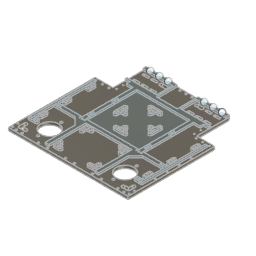
Chassis-200x200x8mm (Autodesk Fusion 360 design; units mm, degrees)
part number: 2026-04-02-11-57-34-569
Autodesk Fusion 360 part; units mm, degrees
(part 1 of 2)
sketch "Sketch1" plane through (0, 0, 0) normal (0, 0, 1) x (1, 0, 0)
  line L0 (67.5, 102.5) -> (-72.5, 102.5)
  line L1 (-102.5, 47.5) -> (-102.5, -97.5)
  line L2 (-102.5, -97.5) -> (97.5, -97.5)
  line L3 (97.5, -97.5) -> (97.5, 47.5)
  line L4 (-72.5, 102.5) -> (-72.5, 52.5)
  line L5 (67.5, 102.5) -> (67.5, 52.5)
  line L6 (-65.9, 77.6) -> (-58.1, 77.6)
  line L7 (-65.9, 74.4) -> (-58.1, 74.4)
  line L8 (-51.9, 77.6) -> (-44.1, 77.6)
  line L9 (-51.9, 74.4) -> (-44.1, 74.4)
  arc A0 (-65.9, 77.6) -> (-65.9, 74.4) centre (-65.9, 76) ccw
  arc A1 (-58.1, 74.4) -> (-58.1, 77.6) centre (-58.1, 76) ccw
  arc A2 (-51.9, 77.6) -> (-51.9, 74.4) centre (-51.9, 76) ccw
  arc A3 (-44.1, 74.4) -> (-44.1, 77.6) centre (-44.1, 76) ccw
  arc A4 (-44.1, 90.4) -> (-44.1, 93.6) centre (-44.1, 92) ccw
  line L10 (-51.9, 90.4) -> (-44.1, 90.4)
  line L11 (-51.9, 93.6) -> (-44.1, 93.6)
  arc A5 (-51.9, 93.6) -> (-51.9, 90.4) centre (-51.9, 92) ccw
  line L12 (-65.9, 93.6) -> (-58.1, 93.6)
  arc A6 (-58.1, 90.4) -> (-58.1, 93.6) centre (-58.1, 92) ccw
  line L13 (-65.9, 90.4) -> (-58.1, 90.4)
  arc A7 (-65.9, 93.6) -> (-65.9, 90.4) centre (-65.9, 92) ccw
  line L14 (39.1, 74.4) -> (46.9, 74.4)
  arc A8 (39.1, 77.6) -> (39.1, 74.4) centre (39.1, 76) ccw
  line L15 (39.1, 77.6) -> (46.9, 77.6)
  arc A9 (46.9, 74.4) -> (46.9, 77.6) centre (46.9, 76) ccw
  arc A10 (53.1, 77.6) -> (53.1, 74.4) centre (53.1, 76) ccw
  line L16 (53.1, 74.4) -> (60.9, 74.4)
  line L17 (53.1, 77.6) -> (60.9, 77.6)
  arc A11 (60.9, 74.4) -> (60.9, 77.6) centre (60.9, 76) ccw
  arc A12 (39.1, 93.6) -> (39.1, 90.4) centre (39.1, 92) ccw
  line L18 (39.1, 90.4) -> (46.9, 90.4)
  line L19 (39.1, 93.6) -> (46.9, 93.6)
  arc A13 (46.9, 90.4) -> (46.9, 93.6) centre (46.9, 92) ccw
  line L20 (53.1, 90.4) -> (60.9, 90.4)
  arc A14 (53.1, 93.6) -> (53.1, 90.4) centre (53.1, 92) ccw
  line L21 (53.1, 93.6) -> (60.9, 93.6)
  arc A15 (60.9, 90.4) -> (60.9, 93.6) centre (60.9, 92) ccw
  arc A16 (-37.9, 77.6) -> (-37.9, 74.4) centre (-37.9, 76) ccw
  line L22 (-37.9, 77.6) -> (-30.1, 77.6)
  arc A17 (-30.1, 74.4) -> (-30.1, 77.6) centre (-30.1, 76) ccw
  line L23 (-37.9, 74.4) -> (-30.1, 74.4)
  line L24 (25.1, 77.6) -> (32.9, 77.6)
  arc A18 (32.9, 74.4) -> (32.9, 77.6) centre (32.9, 76) ccw
  line L25 (25.1, 74.4) -> (32.9, 74.4)
  arc A19 (25.1, 77.6) -> (25.1, 74.4) centre (25.1, 76) ccw
  line L26 (-36.9, 94.551) -> (-28.0006, 94.551)
  line L27 (-36.9006, 89.451) -> (-28.0006, 89.451)
  arc A20 (-36.9, 94.551) -> (-36.9006, 89.451) centre (-36.9006, 92.001) ccw
  arc A21 (-28.0006, 89.451) -> (-28.0006, 94.551) centre (-28.0006, 92.001) ccw
  line L28 (23, 94.551) -> (31.8994, 94.551)
  arc A22 (23, 94.551) -> (22.9994, 89.451) centre (22.9994, 92.001) ccw
  line L29 (22.9994, 89.451) -> (31.8994, 89.451)
  arc A23 (31.8994, 89.451) -> (31.8994, 94.551) centre (31.8994, 92.001) ccw
  line L30 (-72.5, 52.5) -> (-72.5, 47.5)
  line L31 (-72.5, 47.5) -> (-102.5, 47.5)
  line L32 (67.5, 52.5) -> (67.5, 47.5)
  line L33 (67.5, 47.5) -> (97.5, 47.5)
  line L34 (97.5, -97.5) -> (-102.5, -97.5)
  line L35 (-102.5, -97.5) -> (-102.5, -92.5)
  line L36 (97.5, -92.5) -> (97.5, -97.5)
  line L37 (75.5, -90.5) -> (45.5, -90.5)
  line L38 (45.5, -90.5) -> (45.5, -40.5)
  line L39 (45.5, -40.5) -> (75.5, -40.5)
  line L40 (75.5, -40.5) -> (75.5, -90.5)
  line L41 (-80.5, -90.5) -> (-50.5, -90.5)
  line L42 (-50.5, -90.5) -> (-50.5, -40.5)
  line L43 (-50.5, -40.5) -> (-80.5, -40.5)
  line L44 (-80.5, -40.5) -> (-80.5, -90.5)
  line L45 (79, -84.449) -> (85.3494, -84.449)
  line L46 (78.9994, -89.549) -> (87.8994, -89.549)
  arc A24 (87.8994, -89.549) -> (90.4494, -86.9852) centre (87.8994, -86.999) ccw
  arc A25 (79, -84.449) -> (78.9994, -89.549) centre (78.9994, -86.999) ccw
  line L47 (-93.0006, -89.549) -> (-84.1006, -89.549)
  line L48 (-90.4506, -84.449) -> (-84.1006, -84.449)
  arc A26 (-84.1006, -89.549) -> (-84.1006, -84.449) centre (-84.1006, -86.999) ccw
  arc A27 (-95.5506, -86.985) -> (-93.0006, -89.549) centre (-93.0006, -86.999) ccw
  line L49 (90.4494, -86.9991) -> (90.4494, -78.099)
  arc A28 (87.8854, -89.549) -> (90.4494, -86.9991) centre (87.8994, -86.9991) ccw
  line L50 (85.3494, -84.449) -> (85.3494, -78.099)
  arc A29 (90.4494, -78.099) -> (85.3494, -78.099) centre (87.8994, -78.099) ccw
  line L51 (-95.5506, -78.099) -> (-95.5506, -86.9991)
  arc A30 (-90.4506, -78.0996) -> (-95.5506, -78.099) centre (-93.0006, -78.099) ccw
  line L52 (-90.4506, -78.0996) -> (-90.4506, -84.449)
  arc A31 (-95.5506, -86.9991) -> (-92.9866, -89.549) centre (-93.0006, -86.9991) ccw
  circle A32 centre (-65.5, -65.5) radius 15
  circle A33 centre (-65.5, -85) radius 2
  circle A34 centre (-65.5, -46) radius 2
  circle A35 centre (60.5, -85) radius 2
  circle A36 centre (60.5, -65.5) radius 15
  circle A37 centre (60.5, -46) radius 2
  line L53 (75.5, -80.5) -> (45.5, -80.5)
  line L54 (75.5, -50.5) -> (45.5, -50.5)
  line L55 (-50.5, -80.5) -> (-80.5, -80.5)
  line L56 (-50.5, -50.5) -> (-80.5, -50.5)
  line L57 (-70.5, 67.5) -> (-72.5, 67.5)
  line L58 (-70.5, 67.5) -> (-64.5, 67.5)
  line L59 (-64.5, 67.5) -> (-62.5, 67.5)
  circle A38 centre (-67.5, 59.5) radius 1.15
  circle A39 centre (-67.5, 48.623) radius 1.15
  circle A40 centre (-67.5, 48.623) radius 1.15
  circle A41 centre (-67.5, 59.5) radius 1.15
  line L60 (-64.5, 67.5) -> (-62.5, 67.5)
  line L61 (-70.5, 67.5) -> (-64.5, 67.5)
  line L62 (-70.5, 67.5) -> (-72.5, 67.5)
  circle A42 centre (62.5, 48.623) radius 1.15
  circle A43 centre (62.5, 59.5) radius 1.15
  line L63 (65.5, 67.5) -> (67.5, 67.5)
  line L64 (59.5, 67.5) -> (65.5, 67.5)
  line L65 (59.5, 67.5) -> (57.5, 67.5)
  circle A44 centre (-86.5, 43.5) radius 1.35
  circle A45 centre (-97.5, 43.5) radius 1.35
  circle A46 centre (-75.5, 43.5) radius 1.35
  circle A47 centre (92.5, 43.5) radius 1.35
  circle A48 centre (70.5, 43.5) radius 1.35
  circle A49 centre (81.5, 43.5) radius 1.35
  line L66 (-2.5, -97.5) -> (-2.5, 102.5)
  circle A50 centre (2.5, 94.5) radius 1.6
  dimension "d64" = 200
  dimension "d104" = 6
  dimension "d107" = 2
  dimension "d110" = 6
  dimension "d111" = 2
  dimension "d121" = 2.7
  dimension "d122" = 2.7
  dimension "d165" = 50
  dimension "d166" = 10
  dimension "d167" = 30
  dimension "d181" = 2.3
  dimension "d237" = 8.9001
  dimension "d238" = 5.1
  constraint horizontal L0
  constraint perpendicular L0 L1
  constraint parallel L0 L2
  constraint parallel L1 L3
  constraint vertical L4
  constraint vertical L5
  constraint tangent L6 A1
  constraint tangent L7 A1
  constraint tangent L8 A3
  constraint tangent L9 A3
  constraint tangent L12 A6
  constraint tangent A6 L13
  constraint tangent A4 L11
  constraint tangent A4 L10
  constraint tangent L15 A9
  constraint tangent L14 A9
  constraint tangent L17 A11
  constraint tangent L16 A11
  constraint tangent L19 A13
  constraint tangent L18 A13
  constraint tangent L21 A15
  constraint tangent L20 A15
  constraint tangent L22 A17
  constraint tangent A17 L23
  constraint tangent L24 A18
  constraint tangent A18 L25
  constraint tangent L26 A21
  constraint horizontal L26
  constraint tangent L27 A21
  constraint tangent L28 A23
  constraint horizontal L28
  constraint tangent L29 A23
  constraint perpendicular L1 L31
  constraint perpendicular L3 L33
  constraint horizontal L34
  constraint vertical L35
  constraint vertical L36
  constraint horizontal L37
  constraint vertical L38
  constraint horizontal L39
  constraint vertical L40
  constraint horizontal L41
  constraint vertical L42
  constraint horizontal L43
  constraint vertical L44
  constraint tangent L45 A24
  constraint tangent L46 A24
  constraint tangent L48 A26
  constraint tangent L47 A26
  constraint tangent L50 A29
  constraint tangent L49 A29
  constraint tangent L52 A31
  constraint tangent L51 A31
  constraint coincident L47 A31.end
  constraint coincident L51 A27.start
  constraint coincident L46 A28.start
  constraint coincident L49 A24.end
  constraint coincident L40 L53.start
  constraint perpendicular L38 L53
  constraint coincident L40 L54.start
  constraint coincident L38 L54.end
  constraint perpendicular L38 L54
  constraint coincident L4 L57.end
  constraint perpendicular L4 L57
  constraint parallel L58 L59
  constraint parallel L60 L61
  constraint midpoint L34 L66.start
  constraint midpoint L0 L66.end
  constraint perpendicular L0 L66
  measures "d64" distance of L2.end L1.end
  measures "d104" distance of L57.start L58.end
  measures "d107" distance of L58.end L59.end
  measures "d110" distance of L57.start L58.end
  measures "d111" distance of L59.end L58.end
  measures "d121" diameter of A46
  measures "d122" diameter of A47
  measures "d165" distance of L41 L43
  measures "d166" distance of L43 L56
  measures "d167" distance of L42 L44
  measures "d181" diameter of A39
  measures "d237" distance of A22.centre A23.centre
  measures "d238" distance of L28 L29
extrude "Extrude1" add sketch "Sketch1" along normal blind 5 contours L0 L2 L3 L5 L32 L33 L34 L36 L66 | L0 L1 L2 L4 L30 L31 L34 L35 L66 | L37 L38 L40 L53 | L40 A36 L53 | L38 A36 L53 | L40 A36 L54 | L38 A36 L54 | L38 L39 L40 L54 | L41 L42 L44 L55 | L44 A32 L55 | L42 A32 L55 | L44 A32 L56 | L42 A32 L56 | L42 L43 L44 L56 | A50 makes body 1
fillet "Fillet1" radius 3 1 edges at (-2.5, 102.5, 0) on bodies 1
sketch "Sketch2" plane through (0, 0, 5) normal (0, 0, 1) x (-1, 0, 0)
  line L0 (-67.5, -102.5) -> (72.5, -102.5)
  line L1 (72.5, -102.5) -> (72.5, -47.5)
  line L2 (102.5, -47.5) -> (102.5, 97.5)
  line L3 (102.5, 97.5) -> (-97.5, 97.5)
  line L4 (-97.5, 97.5) -> (-97.5, -47.5)
  line L5 (-67.5, -47.5) -> (-67.5, -102.5)
  line L6 (72.5, -102.5) -> (22.5, -102.5)
  line L7 (22.5, -102.5) -> (22.5, -97.5)
  line L8 (22.5, -97.5) -> (72.5, -97.5)
  line L9 (72.5, -97.5) -> (72.5, -102.5)
  line L10 (27.5, -67.5) -> (72.5, -67.5)
  line L11 (72.5, -67.5) -> (72.5, -70.5)
  line L12 (-22.5, -67.5) -> (-67.5, -67.5)
  line L13 (-67.5, -67.5) -> (-67.5, -70.5)
  arc A0 (65.9, -77.6) -> (65.9, -74.4) centre (65.9, -76) ccw
  line L14 (65.9, -77.6) -> (58.1, -77.6)
  arc A1 (58.1, -74.4) -> (58.1, -77.6) centre (58.1, -76) ccw
  line L15 (58.1, -74.4) -> (65.9, -74.4)
  arc A2 (-53.1, -93.6) -> (-53.1, -90.4) centre (-53.1, -92) ccw
  line L16 (-53.1, -93.6) -> (-60.9, -93.6)
  arc A3 (-60.9, -90.4) -> (-60.9, -93.6) centre (-60.9, -92) ccw
  line L17 (-60.9, -90.4) -> (-53.1, -90.4)
  arc A4 (65.9, -93.6) -> (65.9, -90.4) centre (65.9, -92) ccw
  line L18 (65.9, -93.6) -> (58.1, -93.6)
  arc A5 (58.1, -90.4) -> (58.1, -93.6) centre (58.1, -92) ccw
  line L19 (58.1, -90.4) -> (65.9, -90.4)
  arc A6 (-39.1, -77.6) -> (-39.1, -74.4) centre (-39.1, -76) ccw
  line L20 (-39.1, -77.6) -> (-46.9, -77.6)
  arc A7 (-46.9, -74.4) -> (-46.9, -77.6) centre (-46.9, -76) ccw
  line L21 (-46.9, -74.4) -> (-39.1, -74.4)
  arc A8 (-53.1, -77.6) -> (-53.1, -74.4) centre (-53.1, -76) ccw
  line L22 (-53.1, -77.6) -> (-60.9, -77.6)
  arc A9 (-60.9, -74.4) -> (-60.9, -77.6) centre (-60.9, -76) ccw
  line L23 (-60.9, -74.4) -> (-53.1, -74.4)
  arc A10 (51.9, -93.6) -> (51.9, -90.4) centre (51.9, -92) ccw
  line L24 (51.9, -93.6) -> (44.1, -93.6)
  arc A11 (44.1, -90.4) -> (44.1, -93.6) centre (44.1, -92) ccw
  line L25 (44.1, -90.4) -> (51.9, -90.4)
  arc A12 (51.9, -77.6) -> (51.9, -74.4) centre (51.9, -76) ccw
  line L26 (51.9, -77.6) -> (44.1, -77.6)
  arc A13 (44.1, -74.4) -> (44.1, -77.6) centre (44.1, -76) ccw
  line L27 (44.1, -74.4) -> (51.9, -74.4)
  arc A14 (-39.1, -93.6) -> (-39.1, -90.4) centre (-39.1, -92) ccw
  line L28 (-39.1, -93.6) -> (-46.9, -93.6)
  arc A15 (-46.9, -90.4) -> (-46.9, -93.6) centre (-46.9, -92) ccw
  line L29 (-46.9, -90.4) -> (-39.1, -90.4)
  arc A16 (-25.1, -77.6) -> (-25.1, -74.4) centre (-25.1, -76) ccw
  line L30 (-25.1, -77.6) -> (-32.9, -77.6)
  arc A17 (-32.9, -74.4) -> (-32.9, -77.6) centre (-32.9, -76) ccw
  line L31 (-32.9, -74.4) -> (-25.1, -74.4)
  arc A18 (37.9, -77.6) -> (37.9, -74.4) centre (37.9, -76) ccw
  line L32 (37.9, -77.6) -> (30.1, -77.6)
  arc A19 (30.1, -74.4) -> (30.1, -77.6) centre (30.1, -76) ccw
  line L33 (30.1, -74.4) -> (37.9, -74.4)
  line L34 (-67.5, -102.5) -> (-17.5, -102.5)
  line L35 (-17.5, -102.5) -> (-17.5, -97.5)
  line L36 (-17.5, -97.5) -> (-67.5, -97.5)
  line L37 (-67.5, -97.5) -> (-67.5, -102.5)
  line L38 (72.5, -47.5) -> (102.5, -47.5)
  line L39 (-97.5, -47.5) -> (-67.5, -47.5)
  arc A20 (-23, -94.551) -> (-22.9994, -89.451) centre (-22.9994, -92.001) ccw
  line L40 (-23, -94.551) -> (-31.8994, -94.551)
  arc A21 (-31.8994, -89.451) -> (-31.8994, -94.551) centre (-31.8994, -92.001) ccw
  line L41 (-31.8994, -89.451) -> (-22.9994, -89.451)
  arc A22 (36.9, -94.551) -> (36.9006, -89.451) centre (36.9006, -92.001) ccw
  line L42 (36.9, -94.551) -> (28.0006, -94.551)
  arc A23 (28.0006, -89.451) -> (28.0006, -94.551) centre (28.0006, -92.001) ccw
  line L43 (28.0006, -89.451) -> (36.9006, -89.451)
  circle A24 centre (65.5, 85) radius 2
  circle A25 centre (-60.5, 46) radius 2
  circle A26 centre (-60.5, 65.5) radius 15
  arc A27 (-79, 84.449) -> (-78.9994, 89.549) centre (-78.9994, 86.999) ccw
  line L44 (-79, 84.449) -> (-85.3494, 84.449)
  line L45 (-85.3494, 84.449) -> (-85.3494, 78.099)
  arc A28 (-90.4494, 78.099) -> (-85.3494, 78.099) centre (-87.8994, 78.099) ccw
  line L46 (-90.4494, 78.099) -> (-90.4494, 86.9852)
  arc A29 (-89.7213, 88.7832) -> (-90.4494, 86.9852) centre (-87.8994, 86.999) ccw
  arc A30 (-87.8854, 89.549) -> (-89.7213, 88.7832) centre (-87.8994, 86.9991) ccw
  line L47 (-87.8854, 89.549) -> (-78.9994, 89.549)
  circle A31 centre (-60.5, 85) radius 2
  circle A32 centre (65.5, 46) radius 2
  circle A33 centre (65.5, 65.5) radius 15
  arc A34 (90.4506, 78.0996) -> (95.5506, 78.099) centre (93.0006, 78.099) ccw
  line L48 (90.4506, 78.0996) -> (90.4506, 84.449)
  line L49 (90.4506, 84.449) -> (84.1006, 84.449)
  arc A35 (84.1006, 89.549) -> (84.1006, 84.449) centre (84.1006, 86.999) ccw
  line L50 (84.1006, 89.549) -> (92.9866, 89.549)
  arc A36 (94.8063, 88.7996) -> (92.9866, 89.549) centre (93.0006, 86.9991) ccw
  arc A37 (95.5506, 86.985) -> (94.8063, 88.7996) centre (93.0006, 86.999) ccw
  line L51 (95.5506, 86.985) -> (95.5506, 78.099)
  circle A38 centre (90, -32) radius 1.15
  circle A39 centre (90, 8) radius 1.15
  circle A40 centre (67.5, -59.5) radius 1.15
  circle A41 centre (67.5, -48.623) radius 1.15
  circle A42 centre (-62.5, -48.623) radius 1.15
  circle A43 centre (-62.5, -59.5) radius 1.15
  circle A44 centre (75.5, -43.5) radius 1.35
  circle A45 centre (97.5, -43.5) radius 1.35
  circle A46 centre (86.5, -43.5) radius 1.35
  circle A47 centre (-81.5, -43.5) radius 1.35
  circle A48 centre (-92.5, -43.5) radius 1.35
  circle A49 centre (-70.5, -43.5) radius 1.35
  line L52 (72.5, -67.5) -> (64.5, -67.5)
  line L53 (64.5, -67.5) -> (64.5, -40.6151)
  line L54 (64.5, -40.6151) -> (102.5, -40.6151)
  line L55 (-67.5, -67.5) -> (-59.5, -67.5)
  line L56 (-59.5, -67.5) -> (-59.5, -40.6151)
  line L57 (-59.5, -40.6151) -> (-97.5, -40.6151)
  circle A50 centre (90, -32) radius 1.15
  circle A51 centre (90, -24) radius 1.15
  circle A52 centre (90, 16) radius 1.15
  arc A53 (87.0072, -31.7917) -> (93, -32) centre (90, -32) ccw
  arc A54 (87.0072, -31.7917) -> (93, -32) centre (90, -32) ccw
  arc A55 (93, -24) -> (87, -24.0028) centre (90, -24) ccw
  line L58 (93, -32) -> (93, -24)
  line L59 (87.0072, -31.7917) -> (87, -24.0028)
  circle A56 centre (89.9963, -28) radius 1.4
  line L60 (87.0106, 8.0515) -> (87, 15.996)
  line L61 (93, 8) -> (93, 16)
  circle A57 centre (90, 12) radius 1.4
  arc A58 (87.0104, 8.2491) -> (93, 8) centre (90, 8) ccw
  arc A59 (87.0104, 8.2491) -> (93, 8) centre (90, 8) ccw
  arc A60 (93, 16) -> (87, 15.996) centre (90, 16) ccw
  line L62 (87.0072, -31.7917) -> (87, -24.0028)
  arc A61 (87.0072, -31.7917) -> (93, -32) centre (90, -32) ccw
  line L63 (93, -32) -> (93, -24)
  arc A62 (93, -24) -> (87, -24.0028) centre (90, -24) ccw
  circle A63 centre (90, -24) radius 1.15
  circle A64 centre (89.9963, -28) radius 1.4
  circle A65 centre (90, -32) radius 1.15
  arc A66 (87.0104, 8.2491) -> (93, 8) centre (90, 8) ccw
  line L64 (93, 8) -> (93, 16)
  circle A67 centre (90, 16) radius 1.15
  circle A68 centre (90, 12) radius 1.4
  circle A69 centre (90, 8) radius 1.15
  arc A70 (93, 16) -> (87, 15.996) centre (90, 16) ccw
  line L65 (87.0106, 8.0515) -> (87, 15.996)
  line L66 (47.0072, -31.7917) -> (47, -24.0028)
  arc A71 (47.0072, -31.7917) -> (53, -32) centre (50, -32) ccw
  line L67 (53, -32) -> (53, -24)
  arc A72 (53, -24) -> (47, -24.0028) centre (50, -24) ccw
  circle A73 centre (50, -24) radius 1.15
  circle A74 centre (49.9963, -28) radius 1.4
  circle A75 centre (50, -32) radius 1.15
  line L68 (47.0106, 8.0515) -> (47, 15.996)
  arc A76 (47.0104, 8.2491) -> (53, 8) centre (50, 8) ccw
  line L69 (53, 8) -> (53, 16)
  arc A77 (53, 16) -> (47, 15.996) centre (50, 16) ccw
  circle A78 centre (50, 8) radius 1.15
  circle A79 centre (50, 12) radius 1.4
  circle A80 centre (50, 16) radius 1.15
  line L70 (-87.9928, -31.7917) -> (-88, -24.0028)
  arc A81 (-87.9928, -31.7917) -> (-82, -32) centre (-85, -32) ccw
  line L71 (-82, -32) -> (-82, -24)
  arc A82 (-82, -24) -> (-88, -24.0028) centre (-85, -24) ccw
  circle A83 centre (-85, -24) radius 1.15
  circle A84 centre (-85.0037, -28) radius 1.4
  circle A85 centre (-85, -32) radius 1.15
  line L72 (-87.9894, 8.0515) -> (-88, 15.996)
  arc A86 (-87.9896, 8.2491) -> (-82, 8) centre (-85, 8) ccw
  line L73 (-82, 8) -> (-82, 16)
  arc A87 (-82, 16) -> (-88, 15.996) centre (-85, 16) ccw
  circle A88 centre (-85, 8) radius 1.15
  circle A89 centre (-85, 12) radius 1.4
  circle A90 centre (-85, 16) radius 1.15
  arc A91 (-47.9928, -31.7917) -> (-42, -32) centre (-45, -32) ccw
  circle A92 centre (-45, -32) radius 1.15
  line L74 (-42, -32) -> (-42, -24)
  line L75 (-47.9928, -31.7917) -> (-48, -24.0028)
  circle A93 centre (-45.0037, -28) radius 1.4
  circle A94 centre (-45, -24) radius 1.15
  arc A95 (-42, -24) -> (-48, -24.0028) centre (-45, -24) ccw
  arc A96 (-47.9896, 8.2491) -> (-42, 8) centre (-45, 8) ccw
  line L76 (-47.9894, 8.0515) -> (-48, 15.996)
  arc A97 (-42, 16) -> (-48, 15.996) centre (-45, 16) ccw
  line L77 (-42, 8) -> (-42, 16)
  circle A98 centre (-45, 12) radius 1.4
  circle A99 centre (-45, 16) radius 1.15
  circle A100 centre (-45, 8) radius 1.15
  line L78 (-35, -59) -> (40, -59)
  line L79 (40, -59) -> (40, 21)
  line L80 (40, 21) -> (-35, 21)
  line L81 (-35, 21) -> (-35, -59)
  line L82 (64, -67.5) -> (64, -61.5)
  line L83 (64, -61.5) -> (-59, -61.5)
  line L84 (-59, -61.5) -> (-59, -67.5)
  line L85 (27.5, -67.5) -> (-22.5, -67.5)
  line L86 (102.5, -40.6151) -> (97.5, -40.6151)
  line L87 (97.5, -40.6151) -> (97.5, 91.5)
  line L88 (102.5, 97.5) -> (102.5, -40.6151)
  line L89 (-97.5, -40.6151) -> (-92.5, -40.6151)
  line L90 (-92.5, -40.6151) -> (-92.5, 91.5)
  line L91 (-97.5, 97.5) -> (-97.5, -40.6151)
  line L92 (94.5, 29.5) -> (59, 29.5)
  line L93 (47, 23.5) -> (47, -61.5)
  line L94 (47, -61.5) -> (53, -61.5)
  line L95 (53, -61.5) -> (53, 23.5)
  line L96 (-89.5, 29.5) -> (-54, 29.5)
  line L97 (-42, 23.5) -> (-42, -61.5)
  line L98 (-42, -61.5) -> (-48, -61.5)
  line L99 (-48, -61.5) -> (-48, 23.5)
  line L100 (41, 29.5) -> (-36, 29.5)
  line L101 (94.5, 23.5) -> (53, 23.5)
  line L102 (47, 23.5) -> (-42, 23.5)
  line L103 (-48, 23.5) -> (-89.5, 23.5)
  line L104 (22.5, -102.5) -> (20, -102.5)
  line L105 (20, -102.5) -> (20, -67.5)
  line L106 (20, -67.5) -> (22.5, -67.5)
  line L107 (22.5, -67.5) -> (22.5, -102.5)
  line L108 (-17.5, -102.5) -> (-15, -102.5)
  line L109 (-15, -102.5) -> (-15, -67.5)
  line L110 (-15, -67.5) -> (-17.5, -67.5)
  line L111 (-17.5, -67.5) -> (-17.5, -102.5)
  line L112 (22.5, -70.5) -> (72.5, -70.5)
  line L113 (-17.5, -70.5) -> (-67.5, -70.5)
  line L114 (97.5, 91.5) -> (-92.5, 91.5)
  line L115 (47, 41.5) -> (47, 91.5)
  line L116 (41, 29.5) -> (41, 91.5)
  line L117 (50.5, 40.5) -> (80.5, 40.5)
  line L118 (80.5, 40.5) -> (80.5, 90.5)
  line L119 (80.5, 90.5) -> (50.5, 90.5)
  line L120 (50.5, 90.5) -> (50.5, 40.5)
  line L121 (50.5, 40.5) -> (80.5, 90.5) construction
  line L122 (80.5, 40.5) -> (50.5, 90.5) construction
  line L123 (59, 29.5) -> (47, 41.5)
  line L124 (59, 29.5) -> (75.9706, 29.5) construction
  line L125 (-42, 41.5) -> (-42, 91.5)
  line L126 (-36, 91.5) -> (-36, 29.5)
  line L127 (-54, 29.5) -> (-42, 41.5)
  line L128 (87.0072, -31.7917) -> (87, -24.0028)
  arc A101 (87.0072, -31.7917) -> (93, -32) centre (90, -32) ccw
  line L129 (93, -32) -> (93, -24)
  arc A102 (93, -24) -> (87, -24.0028) centre (90, -24) ccw
  circle A103 centre (89.9963, -28) radius 1.4
  circle A104 centre (90, -32) radius 1.15
  circle A105 centre (90, -24) radius 1.15
  line L130 (87.0106, 8.0515) -> (87, 15.996)
  arc A106 (87.0104, 8.2491) -> (93, 8) centre (90, 8) ccw
  line L131 (93, 8) -> (93, 16)
  arc A107 (93, 16) -> (87, 15.996) centre (90, 16) ccw
  circle A108 centre (90, 16) radius 1.15
  circle A109 centre (90, 12) radius 1.4
  circle A110 centre (90, 8) radius 1.15
  line L132 (87.0106, 48.0515) -> (87, 55.996)
  arc A111 (87.0104, 48.2491) -> (93, 48) centre (90, 48) ccw
  line L133 (93, 48) -> (93, 56)
  circle A112 centre (90, 52) radius 1.4
  arc A113 (93, 56) -> (87, 55.996) centre (90, 56) ccw
  circle A114 centre (90, 48) radius 1.15
  circle A115 centre (90, 56) radius 1.15
  line L134 (-87.9894, 48.0515) -> (-88, 55.996)
  arc A116 (-87.9896, 48.2491) -> (-82, 48) centre (-85, 48) ccw
  line L135 (-82, 48) -> (-82, 56)
  circle A117 centre (-85, 52) radius 1.4
  arc A118 (-82, 56) -> (-88, 55.996) centre (-85, 56) ccw
  circle A119 centre (-85, 48) radius 1.15
  circle A120 centre (-85, 56) radius 1.15
  line L136 (87.0106, 8.0515) -> (87, 15.996)
  arc A121 (87.0104, 8.2491) -> (93, 8) centre (90, 8) ccw
  line L137 (93, 8) -> (93, 16)
  circle A122 centre (90, 12) radius 1.4
  arc A123 (93, 16) -> (87, 15.996) centre (90, 16) ccw
  circle A124 centre (90, 8) radius 1.15
  circle A125 centre (90, 16) radius 1.15
  line L138 (93.9776, 23.529) -> (86.0331, 23.5184)
  arc A126 (93.7799, 23.5288) -> (94.029, 29.5184) centre (94.029, 26.5184) ccw
  line L139 (94.029, 29.5184) -> (86.029, 29.5184)
  circle A127 centre (90.029, 26.5184) radius 1.4
  arc A128 (86.029, 29.5184) -> (86.0331, 23.5184) centre (86.029, 26.5184) ccw
  circle A129 centre (94.029, 26.5184) radius 1.15
  circle A130 centre (86.029, 26.5184) radius 1.15
  line L140 (87.0106, 8.0515) -> (87, 15.996)
  arc A131 (87.0104, 8.2491) -> (93, 8) centre (90, 8) ccw
  line L141 (93, 8) -> (93, 16)
  circle A132 centre (90, 12) radius 1.4
  arc A133 (93, 16) -> (87, 15.996) centre (90, 16) ccw
  circle A134 centre (90, 8) radius 1.15
  circle A135 centre (90, 16) radius 1.15
  line L142 (86, 63.5) -> (94, 63.5)
  circle A136 centre (90, 66.5) radius 1.4
  arc A137 (94, 63.5) -> (93.996, 69.5) centre (94, 66.5) ccw
  arc A138 (86.2491, 69.4896) -> (86, 63.5) centre (86, 66.5) ccw
  line L143 (86.0515, 69.4894) -> (93.996, 69.5)
  circle A139 centre (86, 66.5) radius 1.15
  circle A140 centre (94, 66.5) radius 1.15
  line L144 (46, 23.5) -> (54, 23.5)
  circle A141 centre (50, 26.5) radius 1.4
  arc A142 (54, 23.5) -> (53.996, 29.5) centre (54, 26.5) ccw
  arc A143 (46.2491, 29.4896) -> (46, 23.5) centre (46, 26.5) ccw
  line L145 (46.0515, 29.4894) -> (53.996, 29.5)
  circle A144 centre (46, 26.5) radius 1.15
  circle A145 centre (54, 26.5) radius 1.15
  line L146 (-82, 48) -> (-82, 56)
  arc A146 (-87.9896, 48.2491) -> (-82, 48) centre (-85, 48) ccw
  line L147 (-87.9894, 48.0515) -> (-88, 55.996)
  arc A147 (-82, 56) -> (-88, 55.996) centre (-85, 56) ccw
  circle A148 centre (-85, 56) radius 1.15
  circle A149 centre (-85, 52) radius 1.4
  circle A150 centre (-85, 48) radius 1.15
  line L148 (-81, 29.5) -> (-89, 29.5)
  arc A151 (-81.2491, 23.5104) -> (-81, 29.5) centre (-81, 26.5) ccw
  line L149 (-81.0515, 23.5106) -> (-88.996, 23.5)
  arc A152 (-89, 29.5) -> (-88.996, 23.5) centre (-89, 26.5) ccw
  circle A153 centre (-89, 26.5) radius 1.15
  circle A154 centre (-85, 26.5) radius 1.4
  circle A155 centre (-81, 26.5) radius 1.15
  line L150 (-89, 63.5) -> (-81, 63.5)
  arc A156 (-88.7509, 69.4896) -> (-89, 63.5) centre (-89, 66.5) ccw
  line L151 (-88.9485, 69.4894) -> (-81.004, 69.5)
  arc A157 (-81, 63.5) -> (-81.004, 69.5) centre (-81, 66.5) ccw
  circle A158 centre (-81, 66.5) radius 1.15
  circle A159 centre (-85, 66.5) radius 1.4
  circle A160 centre (-89, 66.5) radius 1.15
  line L152 (-49, 23.5) -> (-41, 23.5)
  arc A161 (-48.7509, 29.4896) -> (-49, 23.5) centre (-49, 26.5) ccw
  line L153 (-48.9485, 29.4894) -> (-41.004, 29.5)
  arc A162 (-41, 23.5) -> (-41.004, 29.5) centre (-41, 26.5) ccw
  circle A163 centre (-41, 26.5) radius 1.15
  circle A164 centre (-45, 26.5) radius 1.4
  circle A165 centre (-49, 26.5) radius 1.15
  line L154 (-82, 48) -> (-82, 56)
  arc A166 (-87.9896, 48.2491) -> (-82, 48) centre (-85, 48) ccw
  line L155 (-87.9894, 48.0515) -> (-88, 55.996)
  arc A167 (-82, 56) -> (-88, 55.996) centre (-85, 56) ccw
  circle A168 centre (-85, 56) radius 1.15
  circle A169 centre (-85, 52) radius 1.4
  circle A170 centre (-85, 48) radius 1.15
  line L156 (-88.9485, 69.4894) -> (-92.5, 69.4894)
  line L157 (-89, 63.5) -> (-92.5, 63.5)
  line L158 (93.996, 69.5) -> (97.5, 69.5047)
  line L159 (94, 63.5) -> (97.5, 63.5)
  line L160 (-92.5, -40.1151) -> (-89.5, -40.1151)
  line L161 (-89.5, -40.1151) -> (-89.5, 23.542)
  line L162 (-89.5, 29.458) -> (-89.5, 63.5)
  line L163 (93.4529, -40.6151) -> (93.4529, -40.1151)
  line L164 (97.5, -40.1151) -> (94.5, -40.1151)
  line L165 (94.5, -40.1151) -> (94.5, 23.5556)
  line L166 (94.5, 29.4812) -> (94.5, 63.5)
  line L167 (38, 34) -> (38, 42)
  arc A171 (38, 42) -> (32, 41.996) centre (35, 42) ccw
  circle A172 centre (35, 42) radius 1.15
  circle A173 centre (35, 38) radius 1.4
  line L168 (87.0106, 48.0515) -> (87, 55.996)
  arc A174 (87.0104, 48.2491) -> (93, 48) centre (90, 48) ccw
  line L169 (93, 48) -> (93, 56)
  arc A175 (93, 56) -> (87, 55.996) centre (90, 56) ccw
  circle A176 centre (90, 56) radius 1.15
  circle A177 centre (90, 52) radius 1.4
  circle A178 centre (90, 48) radius 1.15
  line L170 (27, 31) -> (35, 31)
  arc A179 (27.2491, 36.9896) -> (27, 31) centre (27, 34) ccw
  circle A180 centre (27, 34) radius 1.15
  circle A181 centre (31, 34) radius 1.4
  circle A182 centre (35, 34) radius 1.15
  line L171 (32.0067, 36.996) -> (32, 41.996)
  line L172 (27.0515, 36.9894) -> (32.0067, 36.996)
  arc A183 (35, 31) -> (38, 34.0027) centre (35, 34) ccw
  arc A184 (35, 37) -> (34.996, 37) centre (35, 34) ccw
  line L173 (-33, 42) -> (-33, 34)
  arc A185 (-33, 34) -> (-29.9973, 31) centre (-30, 34) ccw
  line L174 (-30, 31) -> (-22, 31)
  arc A186 (-22, 31) -> (-22.004, 37) centre (-22, 34) ccw
  line L175 (-27.004, 36.9933) -> (-22.004, 37)
  line L176 (-27.0106, 41.9485) -> (-27.004, 36.9933)
  arc A187 (-27.0104, 41.7509) -> (-33, 42) centre (-30, 42) ccw
  circle A188 centre (-30, 42) radius 1.15
  circle A189 centre (-30, 38) radius 1.4
  circle A190 centre (-30, 34) radius 1.15
  circle A191 centre (-26, 34) radius 1.4
  circle A192 centre (-22, 34) radius 1.15
  line L177 (38, 78) -> (38, 86)
  arc A193 (38, 86) -> (34.9973, 89) centre (35, 86) ccw
  line L178 (35, 89) -> (27, 89)
  arc A194 (27, 89) -> (27.004, 83) centre (27, 86) ccw
  line L179 (32.004, 83.0067) -> (27.004, 83)
  line L180 (32.0106, 78.0515) -> (32.004, 83.0067)
  arc A195 (32.0104, 78.2491) -> (38, 78) centre (35, 78) ccw
  circle A196 centre (35, 78) radius 1.15
  circle A197 centre (35, 82) radius 1.4
  circle A198 centre (35, 86) radius 1.15
  circle A199 centre (31, 86) radius 1.4
  circle A200 centre (27, 86) radius 1.15
  line L181 (-22, 89) -> (-30, 89)
  arc A201 (-30, 89) -> (-33, 85.9973) centre (-30, 86) ccw
  line L182 (-33, 86) -> (-33, 78)
  arc A202 (-33, 78) -> (-27, 78.004) centre (-30, 78) ccw
  line L183 (-27.0067, 83.004) -> (-27, 78.004)
  line L184 (-22.0515, 83.0106) -> (-27.0067, 83.004)
  arc A203 (-22.2491, 83.0104) -> (-22, 89) centre (-22, 86) ccw
  circle A204 centre (-22, 86) radius 1.15
  circle A205 centre (-26, 86) radius 1.4
  circle A206 centre (-30, 86) radius 1.15
  circle A207 centre (-30, 82) radius 1.4
  circle A208 centre (-30, 78) radius 1.15
  line L185 (-19.0017, 34.1) -> (24.0017, 34.1)
  line L186 (-30, 75) -> (-30, 45)
  line L187 (24.0017, 85.9) -> (-19.0017, 85.9)
  line L188 (35, 45) -> (35, 75)
  circle A209 centre (100, 29.4184) radius 1.35
  circle A210 centre (100, 9.4184) radius 1.35
  circle A211 centre (100, 49.4184) radius 1.35
  circle A212 centre (100, -10.5816) radius 1.35
  circle A213 centre (-95, -10.5816) radius 1.35
  circle A214 centre (-95, 9.4184) radius 1.35
  circle A215 centre (-95, 29.4184) radius 1.35
  circle A216 centre (-95, 49.4184) radius 1.35
  line L189 (-15, -96.5) -> (20, -96.5)
  circle A217 centre (2.5, -99.5) radius 1.6
  circle A218 centre (-7.5, -99.5) radius 1.6
  circle A219 centre (12.5, -99.5) radius 1.6
  circle A220 centre (-5, 94.5) radius 1.6
  circle A221 centre (10, 94.5) radius 1.6
  circle A222 centre (10, 94.5) radius 1.6
  circle A223 centre (-87.5, 94.5) radius 1.6
  circle A224 centre (92.5, 94.5) radius 1.6
  circle A225 centre (82.5, 94.5) radius 1.6
  circle A226 centre (-77.5, 94.5) radius 1.6
  circle A227 centre (-95, 84) radius 1.35
  circle A228 centre (-95, 93) radius 1.35
  circle A229 centre (100, 93) radius 1.35
  circle A230 centre (100, 84) radius 1.35
  arc A231 (-87.9928, -31.7917) -> (-82, -32) centre (-85, -32) ccw
  line L190 (-82, -32) -> (-82, -24)
  arc A232 (-82, -24) -> (-88, -24.0028) centre (-85, -24) ccw
  line L191 (-87.9928, -31.7917) -> (-88, -24.0028)
  line L192 (5.5, -45) -> (5.5, -40)
  arc A233 (5.5, -40) -> (-0.5, -40.004) centre (2.5, -40) ccw
  circle A234 centre (2.5, -44) radius 1.4
  circle A235 centre (2.5, -40) radius 1.15
  arc A236 (-5.5, -45) -> (-5.496, -51) centre (-5.5, -48) ccw
  line L193 (-0.4933, -45) -> (-5.5, -45)
  circle A237 centre (-1.5, -48) radius 1.4
  circle A238 centre (-5.5, -48) radius 1.15
  line L194 (-0.4933, -45) -> (-0.5, -40.004)
  arc A239 (10.2509, -50.9896) -> (10.5, -45) centre (10.5, -48) ccw
  circle A240 centre (10.5, -48) radius 1.15
  circle A241 centre (6.5, -48) radius 1.4
  circle A242 centre (2.5, -48) radius 1.15
  line L195 (10.5, -45) -> (5.5, -45)
  line L196 (10.2509, -50.9896) -> (-5.496, -51)
  line L197 (10.2509, -50.9896) -> (-5.496, -51)
  arc A243 (10.2509, -50.9896) -> (10.5, -45) centre (10.5, -48) ccw
  line L198 (10.5, -45) -> (5.5, -45)
  line L199 (5.5, -45) -> (5.5, -40)
  arc A244 (5.5, -40) -> (-0.5, -40.004) centre (2.5, -40) ccw
  line L200 (-0.4933, -45) -> (-0.5, -40.004)
  arc A245 (-5.5, -45) -> (-5.496, -51) centre (-5.5, -48) ccw
  line L201 (-0.4933, -45) -> (-5.5, -45)
  circle A246 centre (10.5, -48) radius 1.15
  circle A247 centre (6.5, -48) radius 1.4
  circle A248 centre (2.5, -48) radius 1.15
  circle A249 centre (-1.5, -48) radius 1.4
  circle A250 centre (-5.5, -48) radius 1.15
  circle A251 centre (2.5, -44) radius 1.4
  circle A252 centre (2.5, -40) radius 1.15
  arc A253 (-29.4896, -26.7509) -> (-23.5, -27) centre (-26.5, -27) ccw
  line L202 (-23.5, -27) -> (-23.5, -22)
  line L203 (-23.5, -22) -> (-18.5, -22)
  arc A254 (-18.5, -22) -> (-18.504, -16) centre (-18.5, -19) ccw
  line L204 (-23.5, -16.0067) -> (-18.504, -16)
  line L205 (-23.5, -16.0067) -> (-23.5, -11)
  arc A255 (-23.5, -11) -> (-29.5, -11.004) centre (-26.5, -11) ccw
  line L206 (-29.4896, -26.7509) -> (-29.5, -11.004)
  circle A256 centre (-26.5, -27) radius 1.15
  circle A257 centre (-26.5, -23) radius 1.4
  circle A258 centre (-26.5, -19) radius 1.15
  circle A259 centre (-26.5, -15) radius 1.4
  circle A260 centre (-26.5, -11) radius 1.15
  circle A261 centre (-22.5, -19) radius 1.4
  circle A262 centre (-18.5, -19) radius 1.15
  arc A263 (-5.2509, 12.9896) -> (-5.5, 7) centre (-5.5, 10) ccw
  line L207 (-5.5, 7) -> (-0.5, 7)
  line L208 (-0.5, 7) -> (-0.5, 2)
  arc A264 (-0.5, 2) -> (5.5, 2.004) centre (2.5, 2) ccw
  line L209 (5.4933, 7) -> (5.5, 2.004)
  line L210 (5.4933, 7) -> (10.5, 7)
  arc A265 (10.5, 7) -> (10.496, 13) centre (10.5, 10) ccw
  line L211 (-5.2509, 12.9896) -> (10.496, 13)
  circle A266 centre (-5.5, 10) radius 1.15
  circle A267 centre (-1.5, 10) radius 1.4
  circle A268 centre (2.5, 10) radius 1.15
  circle A269 centre (6.5, 10) radius 1.4
  circle A270 centre (10.5, 10) radius 1.15
  circle A271 centre (2.5, 6) radius 1.4
  circle A272 centre (2.5, 2) radius 1.15
  arc A273 (34.4896, -11.2491) -> (28.5, -11) centre (31.5, -11) ccw
  line L212 (28.5, -11) -> (28.5, -16)
  line L213 (28.5, -16) -> (23.5, -16)
  arc A274 (23.5, -16) -> (23.504, -22) centre (23.5, -19) ccw
  line L214 (28.5, -21.9933) -> (23.504, -22)
  line L215 (28.5, -21.9933) -> (28.5, -27)
  arc A275 (28.5, -27) -> (34.5, -26.996) centre (31.5, -27) ccw
  line L216 (34.4896, -11.2491) -> (34.5, -26.996)
  circle A276 centre (31.5, -11) radius 1.15
  circle A277 centre (31.5, -15) radius 1.4
  circle A278 centre (31.5, -19) radius 1.15
  circle A279 centre (31.5, -23) radius 1.4
  circle A280 centre (31.5, -27) radius 1.15
  circle A281 centre (27.5, -19) radius 1.4
  circle A282 centre (23.5, -19) radius 1.15
  line L217 (2.498, -37) -> (2.502, -1)
  line L218 (-15.5, -18.998) -> (20.5, -19.002)
  line L219 (-8.5, -48.002) -> (-26.5, -48)
  line L220 (-26.502, -8) -> (-26.502, 10)
  line L221 (13.5, 10.002) -> (31.5, 9.9999)
  line L222 (31.502, -30) -> (31.5, -48)
  circle A283 centre (-57.5, -100) radius 1.15
  circle A284 centre (-42.5, -100) radius 1.15
  circle A285 centre (-27.5, -100) radius 1.15
  circle A286 centre (32.5, -100) radius 1.15
  circle A287 centre (47.5, -100) radius 1.15
  circle A288 centre (62.5, -100) radius 1.15
  circle A289 centre (40, 94.5) radius 1.6
  circle A290 centre (55, 94.5) radius 1.6
  circle A291 centre (-35, 94.5) radius 1.6
  circle A292 centre (-50, 94.5) radius 1.6
  point P0 (65.5, 65.5)
  point P1 (90, 48)
  point P2 (-85, 48)
  point P3 (90, 8)
  point P4 (94.029, 26.5184)
  point P5 (90, 8)
  point P6 (35, 34)
  point P7 (90, 48)
  point P8 (-85.0037, -28)
  point P9 (2.5, 10)
  point P10 (2.5, -40)
  point P11 (2.5, -44)
  point P12 (-26.5, -19)
  dimension "d19" = 50
  dimension "d20" = 27
  dimension "d51" = 5
  dimension "d129" = 2.3
  dimension "d132" = 2.8
  dimension "d144" = 6
  dimension "d168" = 30
  dimension "d179" = 0.5
  dimension "d182" = 2.7
  dimension "d191" = 2.7
  dimension "d194" = 3.2
  constraint horizontal L6
  constraint vertical L7
  constraint horizontal L8
  constraint vertical L9
  constraint coincident L0.end L1.start
  constraint horizontal L10
  constraint vertical L11
  constraint coincident L1 L11.end
  constraint horizontal L12
  constraint vertical L13
  constraint coincident L5 L13.end
  constraint horizontal L34
  constraint vertical L35
  constraint horizontal L36
  constraint vertical L37
  constraint coincident L0.start L5.end
  constraint concentric A38 A53
  constraint concentric A39 A59
  constraint perpendicular L11 L52
  constraint perpendicular L52 L53
  constraint coincident L2 L54.end
  constraint perpendicular L2 L54
  constraint perpendicular L13 L55
  constraint perpendicular L12 L56
  constraint coincident L4 L57.end
  constraint perpendicular L4 L57
  constraint concentric A50 A54
  constraint concentric A51 A55
  constraint concentric A52 A60
  constraint tangent A55 L58
  constraint coincident A53 A54.start
  constraint coincident A55 L59.end
  constraint tangent A55 L59
  constraint coincident L59 A53.start
  constraint coincident L59 A55.end
  constraint coincident L60.end A60
  constraint tangent L60 A60
  constraint tangent L61 A60
  constraint coincident L60 A58.start
  constraint coincident L60 A60.end
  constraint concentric A61 A65
  constraint concentric A62 A63
  constraint concentric A67 A70
  constraint tangent L63 A62
  constraint coincident A53.start A61
  constraint coincident A55.end A62
  constraint tangent L62 A62
  constraint coincident A53.start L62
  constraint coincident A55.end L62
  constraint coincident L60.end A70
  constraint tangent A70 L65
  constraint tangent L64 A70
  constraint coincident A58.start L65
  constraint coincident L60.end L65
  constraint concentric A76 A78
  constraint concentric A72 A73
  constraint tangent L67 A72
  constraint concentric A77 A80
  constraint coincident L68.end A77
  constraint tangent L68 A77
  constraint tangent L69 A77
  constraint coincident A77.end L68
  constraint concentric A86 A88
  constraint concentric A82 A83
  constraint tangent L71 A82
  constraint concentric A87 A90
  constraint coincident L72.end A87
  constraint tangent L72 A87
  constraint tangent L73 A87
  constraint coincident A87.end L72
  constraint concentric A96 A100
  constraint concentric A94 A95
  constraint tangent L74 A95
  constraint concentric A97 A99
  constraint coincident L76.end A97
  constraint tangent L76 A97
  constraint tangent A97 L77
  constraint coincident A97.end L76
  constraint horizontal L78
  constraint perpendicular L78 L79
  constraint parallel L78 L80
  constraint parallel L79 L81
  constraint coincident L10 L82.start
  constraint perpendicular L56 L83
  constraint coincident L12 L84.end
  constraint perpendicular L12 L84
  constraint horizontal L86
  constraint vertical L87
  constraint vertical L88
  constraint horizontal L89
  constraint vertical L90
  constraint vertical L91
  constraint perpendicular L90 L101
  constraint perpendicular L87 L92
  constraint vertical L93
  constraint horizontal L94
  constraint vertical L95
  constraint perpendicular L90 L96
  constraint vertical L97
  constraint horizontal L98
  constraint vertical L99
  constraint perpendicular L97 L100
  constraint collinear L101 L102
  constraint collinear L102 L103
  constraint horizontal L104
  constraint vertical L105
  constraint horizontal L106
  constraint vertical L107
  constraint coincident L85 L105.end
  constraint horizontal L108
  constraint vertical L109
  constraint horizontal L110
  constraint vertical L111
  constraint coincident L85 L109.end
  constraint coincident L107 L112.start
  constraint perpendicular L11 L112
  constraint coincident L111 L113.start
  constraint perpendicular L13 L113
  constraint perpendicular L90 L114
  constraint coincident L114 L115.end
  constraint perpendicular L114 L115
  constraint coincident L114 L116.end
  constraint perpendicular L114 L116
  constraint horizontal L117
  constraint perpendicular L117 L118
  constraint parallel L117 L119
  constraint parallel L118 L120
  constraint coincident L121 P0
  constraint coincident L122 P0
  constraint coincident P0 A33.centre
  constraint horizontal L124
  constraint coincident L114 L125.end
  constraint perpendicular L114 L125
  constraint coincident L114 L126.start
  constraint perpendicular L100 L126
  constraint concentric A106 A110
  constraint concentric A101 A104
  constraint concentric A107 A108
  constraint coincident A53.start A101
  constraint coincident A53.start L128
  constraint coincident L60.end A107
  constraint tangent L130 A107
  constraint coincident L60.end L130
  constraint coincident L132.end A113
  constraint tangent L132 A113
  constraint coincident A111.start L132
  constraint coincident A113.end L132
  constraint coincident L134.end A118
  constraint tangent L134 A118
  constraint coincident A116.start L134
  constraint coincident A118.end L134
  constraint coincident L60.end A123
  constraint tangent L136 A123
  constraint coincident A58.start L136
  constraint coincident L60.end L136
  constraint coincident L138.end A128
  constraint tangent L138 A128
  constraint coincident A126.start L138
  constraint coincident A128.end L138
  constraint coincident L60.end A133
  constraint tangent L140 A133
  constraint coincident A58.start L140
  constraint coincident L60.end L140
  constraint coincident L143.end A137
  constraint tangent A137 L143
  constraint coincident A138.start L143
  constraint coincident A137.end L143
  constraint coincident L145.end A142
  constraint tangent A142 L145
  constraint coincident A143.start L145
  constraint coincident A142.end L145
  constraint coincident L134.end A147
  constraint tangent L147 A147
  constraint coincident A116.start L147
  constraint coincident L134.end L147
  constraint coincident L149.end A152
  constraint tangent L149 A152
  constraint coincident A151.start L149
  constraint coincident A152.end L149
  constraint coincident L151.end A157
  constraint tangent L151 A157
  constraint coincident A156.start L151
  constraint coincident A157.end L151
  constraint coincident L153.end A162
  constraint tangent L153 A162
  constraint coincident A161.start L153
  constraint coincident A162.end L153
  constraint coincident L134.end A167
  constraint tangent L155 A167
  constraint coincident A116.start L155
  constraint coincident L134.end L155
  constraint coincident L90 L156.end
  constraint perpendicular L90 L156
  constraint coincident L90 L157.end
  constraint tangent A156 L157
  constraint coincident L87 L158.end
  constraint tangent A137 L158
  constraint coincident L87 L159.end
  constraint tangent A137 L159
  constraint coincident L90 L160.start
  constraint perpendicular L90 L160
  constraint coincident L157 L162.end
  constraint perpendicular L157 L161
  constraint coincident A152 L161.end
  constraint collinear L161 L162
  constraint coincident A152 L162.start
  constraint coincident L162 L96.start
  constraint coincident L161 L103.end
  constraint coincident L54 L163.start
  constraint perpendicular L54 L163
  constraint coincident L87 L164.start
  constraint perpendicular L87 L164
  constraint vertical L165
  constraint coincident L159 L166.end
  constraint coincident L101.start L165
  constraint coincident L92.start L165
  constraint coincident A126 L165.end
  constraint collinear L165 L166
  constraint coincident A126 L166.start
  constraint coincident L171.end A171
  constraint coincident L132.end A175
  constraint tangent L168 A175
  constraint coincident A111.start L168
  constraint coincident L132.end L168
  constraint tangent L172 A183
  constraint coincident A179.start L172
  constraint coincident A184.end L172
  constraint coincident A179 L185.end
  constraint coincident A184.start A183
  constraint coincident L167 A183.end
  constraint concentric A183 A184
  constraint coincident A171 L188.start
  constraint coincident L175.end A186
  constraint tangent A185 L176
  constraint coincident A187.start L176
  constraint coincident A185.end L174
  constraint coincident L179.end A194
  constraint tangent A193 L180
  constraint coincident A195.start L180
  constraint coincident A193.end L178
  constraint coincident L183.end A202
  constraint tangent A201 L184
  constraint coincident A203.start L184
  constraint coincident A201.end L182
  constraint coincident A186 L185.start
  constraint coincident A187 L186.end
  constraint coincident A202 L186.start
  constraint coincident A203 L187.end
  constraint coincident A194 L187.start
  constraint coincident A195 L188.end
  constraint coincident L109 L189.start
  constraint perpendicular L109 L189
  constraint tangent L190 A232
  constraint midpoint A233 L217.start
  constraint midpoint A264 L217.end
  constraint midpoint A254 L218.start
  constraint midpoint A274 L218.end
  constraint perpendicular L217 L218
  constraint midpoint A245 L219.start
  constraint parallel L218 L219
  constraint midpoint A255 L220.start
  constraint vertical L220
  constraint midpoint A265 L221.start
  constraint midpoint A275 L222.start
  measures "d19" distance of L0.end L6.end
  measures "d20" distance of L8.end L11.end
  measures "d51" distance of L0.end L8.end
  measures "d129" diameter of A50
  measures "d132" diameter of A56
  measures "d144" distance of L82.start L82.end
  measures "d168" distance of L118.end L119.end
  measures "d179" distance of L163.start L163.end
  measures "d182" diameter of A209
  measures "d191" diameter of A215
  measures "d194" diameter of A217
extrude "Extrude4" cut sketch "Sketch2" against normal blind 3 contours A38 A50 A65 A104 | A39 A69 A110 A124 A134 | A51 A63 A105 | A52 A67 A108 A125 A135 | A56 A64 A103 | A57 A68 A109 A122 A132 | A73 | A74 | A75 | A78 | A79 | A80 | A83 | A84 | A85 | A88 | A89 | A90 | A92 | A93 | A94 | A98 | A99 | A100 | A117 A149 A169 | A119 A150 A170 | A120 A148 A168 | A127 | A129 | A130 | A136 | A139 | A140 | A141 | A144 | A145 | A153 | A154 | A155 | A158 | A159 | A160 | A163 | A164 | A165 | A172 | A173 | A180 | A181 | A182 | A188 | A189 | A190 | A191 | A192 | A196 | A197 | A198 | A199 | A200 | A204 | A205 | A206 | A207 | A208 | A234 A251 | A235 A252 | A237 A249 | A238 A250 | A240 A246 | A241 A247 | A242 A248 | A256 | A257 | A258 | A259 | A260 | A261 | A262 | A266 | A267 | A268 | A269 | A270 | A271 | A272 | A276 | A277 | A278 | A279 | A280 | A281 | A282 | A283 | A284 | A285 | A286 | A287 | A288 bodies 1
extrude "Extrude5" add sketch "Sketch2" along normal blind 3 separate body contours L0 L5 L34 L35 L36 L37 L111 | L0 L35 L85 L108 L109 L110 L111 | L5 L12 L13 L55 L85 L111 L113 | L0 L7 L85 L104 L105 L106 L107 | L0 L1 L6 L7 L8 L9 L107 | L10 L12 L82 L83 L84 L85 L94 L98 L106 L110 | L1 L10 L11 L52 L85 L107 L112 | A91 L83 L97 L98 L99 | L90 A152 L157 L160 L161 L162 | A91 L74 L75 A95 L97 | L90 A156 L156 L157 | A71 L83 L93 L94 L95 | A95 A96 L97 L99 | L66 A71 L67 A72 L95 | A96 L76 A97 L77 L97 | L150 A156 L151 A157 L156 | A156 L151 L156 | L96 L148 A151 L149 A152 | L87 A126 L159 L164 L165 L166 | A72 A76 L93 L95 | A97 L97 L99 L152 | L92 L96 L100 L101 L102 L103 L114 L115 L116 L123 L125 L126 L127 L138 A126 A128 A142 A143 L145 A151 A161 L153 A162 L165 | L87 A137 L158 L159 | L68 A76 L69 A77 L95 | L102 L103 L152 A161 L153 A162 | A77 L93 L95 L144 | L142 A137 A138 L143 | L101 L102 L144 A142 A143 L145 | L92 L138 A126 A128 | A53 A54 A55 L58 L59 L62 A61 L63 A62 L128 A101 L129 A102 | L60 L61 A58 A59 A60 A66 L64 A70 L65 L130 A106 L131 A107 L136 A121 L137 A123 L140 A131 L141 A133 | L70 A81 L71 A82 A231 L190 A232 L191 | L72 A86 L73 A87 | L132 A111 L133 A113 L168 A174 L169 A175 | L134 A116 L135 A118 L146 A146 L147 A147 L154 A166 L155 A167 | L167 A171 L170 A179 L171 L172 A183 | L177 A193 L178 A194 L179 L180 A195 | L173 A185 L174 A186 L175 L176 A187 | L181 A201 L182 A202 L183 L184 A203 | L192 A233 A236 L193 L194 A239 L195 L196 L197 A243 L198 L199 A244 L200 A245 L201 | A253 L202 L203 A254 L204 L205 A255 L206 | A263 L207 L208 A264 L209 L210 A265 L211 | A273 L212 L213 A274 L214 L215 A275 L216 | A283 | A284 | A285 | A286 | A287 | A288 makes body 2 at (-44.5, 66.5, 5) makes body 3 at (82.5333, -52, 5) makes body 4 at (-92.4667, -52, 5) makes body 5 at (-92.4654, 28, 5) makes body 6 at (-92.4667, -12, 5) makes body 7 at (82.5346, 28, 5) makes body 8 at (82.5333, -12, 5) makes body 9 at (-30.9642, -88.4654, 5) makes body 10 at (-32.5818, -39.1998, 5) makes body 11 at (25.9642, -31.5346, 8) makes body 12 at (27.5818, -80.8002, 8) makes body 13 at (-2.3896, 50.3788, 5) makes body 14 at (-1.3522, -12.4515, 5) makes body 15 at (28.8799, 18.9183, 5) makes body 16 at (-33.8799, 19.0817, 8)